thumbstick (Autodesk Fusion 360 design; units mm, degrees)
Autodesk Fusion 360 part; units mm, degrees
sketch "Sketch1" plane through (0, 0, 0) normal (0, 0, 1) x (1, 0, 0)
  line L0 (0, 0) -> (3, 0)
  line L1 (3, 0) -> (3, 4)
  line L2 (3, 4) -> (0, 4)
  line L3 (0, 4) -> (0, 0)
  line L4 (-1.2, -1.2) -> (4.2, -1.2)
  line L5 (4.2, -1.2) -> (4.2, 5.2)
  line L6 (4.2, 5.2) -> (-1.2, 5.2)
  line L7 (-1.2, 5.2) -> (-1.2, -1.2)
  dimension "d1" = 3
  dimension "d2" = 4
  dimension "d3" = 1.2
  dimension "d4" = 1.2
  dimension "d5" = 1.2
  dimension "d6" = 1.2
  constraint horizontal L0
  constraint vertical L1
  constraint horizontal L2
  constraint vertical L3
  constraint coincident L0.start L3.end
  constraint horizontal L4
  constraint vertical L5
  constraint horizontal L6
  constraint vertical L7
  measures "d1" distance of L0.start L0.end
  measures "d2" distance of L0.end L1.end
  measures "d3" distance of L2 L6
  measures "d4" distance of L1 L5
  measures "d5" distance of L3 L7
  measures "d6" distance of L0 L4
extrude "Extrude1" add sketch "Sketch1" along normal blind 30
